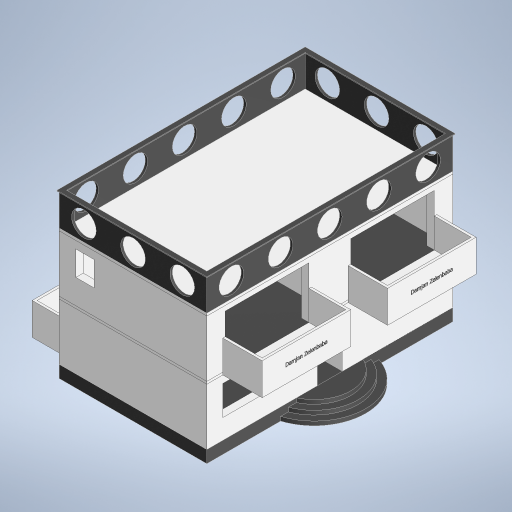
# Autodesk Inventor part: House
Saved by Autodesk Inventor 2024 (Build 280153000, 153)
## iProperties
Created: 2023-06-27
Part Number: House
Material: Generic
Document SubType Name: Modeling
Designer: 69
Density: 1 g/cm^3
Appearance: White
Author: 69
Autodesk Inventor part; units mm, degrees
(part 1 of 3)
ref_plane "YZ Plane" through (0, 0, 0) normal (1, 0, 0) x (0, 1, 0)
ref_plane "XZ Plane" through (0, 0, 0) normal (0, 1, 0) x (-1, 0, 0)
ref_plane "XY Plane" through (0, 0, 0) normal (0, 0, 1) x (1, 0, 0)
sketch "Sketch1" plane through (0, 0, 0) normal (0, 1, 0) x (-1, 0, 0)
  line L0 (3000, 5000) -> (-3000, 5000)
  line L1 (-3000, 5000) -> (-3000, -5000)
  line L2 (-3000, -5000) -> (3000, -5000)
  line L3 (3000, -5000) -> (3000, 5000)
  line L4 (3000, 5000) -> (-3000, -5000) construction
  line L5 (-3000, 5000) -> (3000, -5000) construction
  point P0 (0, 0)
  dimension "d0" = 6000
  dimension "d1" = 10000
  constraints: 12 end point, 2 midpoint, 2 parallel, 1 horizontal, 1 perpendicular
  measures "d0" distance of L2.end L1.end
  measures "d1" distance of L1.end L0.end
extrude "Extrusion1" add sketch "Sketch1" along normal blind 500
sketch "Sketch2" plane through (0, 500, 0) normal (0, 1, 0) x (1, 0, 0)
  line L0 (3000, -5000) -> (3000, 5000) projected
  line L1 (3000, 5000) -> (-3000, 5000) projected
  line L2 (-3000, 5000) -> (-3000, -5000) projected
  line L3 (-3000, -5000) -> (3000, -5000) projected
  line L4 (-2700, -4700) -> (-2700, 4700)
  line L5 (-2700, 4700) -> (2700, 4700)
  line L6 (2700, 4700) -> (2700, -4700)
  line L7 (2700, -4700) -> (-2700, -4700)
  line L8 (2700, 4700) -> (700, 4700)
  line L9 (700, 4700) -> (700, 600)
  line L10 (700, 500) -> (2700, 500)
  line L11 (2700, 500) -> (2700, 4700)
  line L12 (-2700, 4700) -> (600, 4700)
  line L13 (600, 4700) -> (600, 1000)
  line L14 (600, 1000) -> (-2700, 1000)
  line L15 (-2700, 1000) -> (-2700, 4700)
  line L16 (-2700, -4700) -> (-50, -4700)
  line L17 (-50, -4700) -> (-50, -1000)
  line L18 (-50, -1000) -> (-2700, -1000)
  line L19 (-2700, -1000) -> (-2700, -4700)
  line L20 (2700, -4700) -> (50, -4700)
  line L21 (50, -4700) -> (50, -600)
  line L22 (50, -500) -> (2700, -500)
  line L23 (2700, -500) -> (2700, -4700)
  line L24 (-1200, -1000) -> (-1200, 1000)
  line L25 (-2700, -900) -> (-50, -900)
  line L26 (-50, -900) -> (-50, -500)
  line L27 (-50, -500) -> (50, -500)
  line L28 (50, -600) -> (2700, -600)
  line L29 (-2700, 900) -> (600, 900)
  line L30 (600, 900) -> (600, 500)
  line L31 (600, 500) -> (700, 500)
  line L32 (700, 600) -> (2700, 600)
  line L33 (-1200, -50) -> (-1950, -50)
  line L34 (-1950, -50) -> (-1950, 50)
  line L35 (-1950, 50) -> (-1200, 50)
  line L36 (-1200, 50) -> (-1200, -50)
  point P0 (0, 0)
  point P1 (2700, 0)
  point P2 (-2700, 0)
  point P3 (0, -4700)
  point P4 (-1950, 0)
  point P5 (-1200, 0)
  point P6 (-1200, 0)
  point P7 (2700, -600)
  point P8 (50, -4700)
  point P9 (700, 4700)
  point P10 (-2700, -1000)
  point P11 (-50, -4700)
  dimension "d4" = 300
  dimension "d5" = 500
  dimension "d6" = 2000
  dimension "d7" = 1000
  dimension "d8" = 100
  dimension "d9" = 1000
  dimension "d10" = 50
  dimension "d11" = 50
  dimension "d12" = 500
  dimension "d13" = 1500
  dimension "d14" = 100
  dimension "d15" = 100
  dimension "d16" = 100
  dimension "d17" = 100
  dimension "d18" = 100
  dimension "d19" = 100
  dimension "d20" = 2000
  dimension "d21" = 100
  dimension "d22" = 750
  constraints: 66 end point, 13 perpendicular, 10 parallel, 7 point on line, 6 horizontal, 6 midpoint, 2 horizontal alignment, 3 other
  measures "d4" distance between parallel lines of L2 L4
  measures "d5" distance of L10.end point (2700, 0)
  measures "d6" distance of L10.start L10.end
  measures "d7" distance of L14.end point (-2700, 0)
  measures "d8" distance between parallel lines of L9 L13
  measures "d9" distance of point (-2700, 0) L18.end
  measures "d10" distance of point (0, -4700) L16.end
  measures "d11" distance of point (0, -4700) L20.end
  measures "d12" distance of point (2700, 0) L22.end
  measures "d13" distance between parallel lines of L4 L24
  measures "d14" distance between parallel lines of L22 L28
  measures "d15" distance between parallel lines of L21 L26
  measures "d16" distance between parallel lines of L18 L25
  measures "d17" distance between parallel lines of L32 L10
  measures "d18" distance between parallel lines of L9 L30
  measures "d19" distance between parallel lines of L14 L29
  measures "d20" distance between parallel lines of L6 L9
  measures "d21" distance of L33.end L34.end
  measures "d22" distance of L34.end L35.end
extrude "Extrusion2" add sketch "Sketch2" along normal blind 2400 separate body contours L3 L2 L1 L0 | L4 L25 L24 L18 | L17 L18 L24 L25 L26 L27 L22 L6 L28 L21 L7 | L4 L14 L24 L29 | L24 L14 L13 L5 L9 L32 L6 L10 L31 L30 L29 | L33 L34 L35 L24
sketch "Sketch3" plane through (3000, 500, 5000) normal (1, 0, 0) x (0, 0, -1)
  line L0 (0, 0) -> (10000, 0) projected
  line L1 (10000, 0) -> (10000, 2400) projected
  line L2 (0, 2400) -> (10000, 2400) projected
  line L3 (0, 0) -> (0, 2400) projected
  line L4 (0, 0) -> (10000, 0) projected
  line L5 (4500, 0) -> (5500, 0)
  line L6 (5500, 0) -> (5500, 2100)
  line L7 (5500, 2100) -> (4500, 2100)
  line L8 (4500, 2100) -> (4500, 0)
  point P0 (5000, -500)
  point P1 (5000, 0)
  point P2 (4400, 0)
  point P3 (5000, 0)
  dimension "d25" = 2100
  dimension "d26" = 1000
  constraints: 8 end point, 2 midpoint, 2 parallel, 1 coincident, 1 horizontal, 1 horizontal alignment, 1 perpendicular, 1 point on line
  measures "d25" distance of L5.end L6.end
  measures "d26" distance of L6.end L7.end
extrude "Extrusion3" cut sketch "Sketch3" against normal blind 500 contours L8 L7 L6 L0 bodies 2
sketch "Sketch4" plane through (2700, 500, -600) normal (0, 0, -1) x (-1, 0, 0)
  line L0 (1100, 2100) -> (1900, 2100)
  line L1 (1900, 2100) -> (1900, 0)
  line L2 (1900, 0) -> (1100, 0)
  line L3 (1100, 0) -> (1100, 2100)
  line L4 (2000, 0) -> (2000, 2400) projected
  line L5 (0, 0) -> (2000, 0) projected
  point P0 (2700, -500)
  dimension "d29" = 100
  dimension "d30" = 800
  dimension "d31" = 2100
  constraints: 8 end point, 2 parallel, 1 collinear, 1 horizontal, 1 perpendicular
  measures "d29" distance between parallel lines of L4 L1
  measures "d30" distance of L0.start L0.end
  measures "d31" distance of L2.end L0.start
extrude "Extrusion4" cut sketch "Sketch4" against normal blind 200 bodies 2
sketch "Sketch5" plane through (600, 500, -1000) normal (0, 0, -1) x (-1, 0, 0)
  line L0 (100, 2100) -> (900, 2100)
  line L1 (900, 2100) -> (900, 0)
  line L2 (900, 0) -> (100, 0)
  line L3 (100, 0) -> (100, 2100)
  line L4 (0, 0) -> (3300, 0) projected
  line L5 (0, 0) -> (0, 2400) projected
  point P0 (600, -500)
  dimension "d34" = 100
  dimension "d36" = 2100
  dimension "d37" = 800
  constraints: 8 end point, 2 parallel, 1 collinear, 1 horizontal, 1 perpendicular
  measures "d34" distance between parallel lines of L5 L3
  measures "d36" distance of L0.end L1.end
  measures "d37" distance of L0.start L0.end
extrude "Extrusion5" cut sketch "Sketch5" against normal blind 200 bodies 2
sketch "Sketch6" plane through (3000, 500, 500) normal (0, 0, -1) x (-1, 0, 0)
  line L0 (2050, 2100) -> (2850, 2100)
  line L1 (2850, 2100) -> (2850, 0)
  line L2 (2850, 0) -> (2050, 0)
  line L3 (2050, 0) -> (2050, 2100)
  line L4 (0, 0) -> (3050, 0) projected
  line L5 (3050, 0) -> (3050, 2400) projected
  point P0 (3000, -500)
  dimension "d40" = 800
  dimension "d41" = 2100
  dimension "d42" = 200
  constraints: 8 end point, 2 parallel, 1 collinear, 1 horizontal, 1 perpendicular
  measures "d40" distance of L0.start L0.end
  measures "d41" distance of L2.end L0.start
  measures "d42" distance between parallel lines of L5 L1
extrude "Extrusion6" cut sketch "Sketch6" against normal blind 200 bodies 2
sketch "Sketch8" plane through (0, 0, 0) normal (0, 1, 0) x (-1, 0, 0)
  line L0 (-3000, 5000) -> (-3000, -5000) projected
  line L1 (-3000, 5000) -> (-3000, -5000) projected
  arc A0 (-3000, 2000) -> (-3000, -2000) centre (-2359.6876, 0) ccw
  point P0 (0, 0)
  point P1 (-4459.6876, 0)
  point P2 (-3000, 0)
  point P3 (-3000, -2000)
  point P4 (-3000, 2000)
  dimension "d50" = 4000
  dimension "d62" = 2100
  constraints: 3 point on circle, 2 point on line, 1 centre point, 1 horizontal alignment, 1 midpoint
  measures "d50" distance of A0.end A0.start
  measures "d62" radius of A0
extrude "Extrusion8" add sketch "Sketch8" along normal blind 166.66 separate body
sketch "Sketch9" plane through (0, 166.66, 0) normal (0, 1, 0) x (1, 0, 0)
  arc A0 (3000, -2000) -> (3000, 2000) centre (2359.6876, 0) ccw projected
  arc A1 (3000, -1682.2604) -> (3000, 1682.2604) centre (2359.6876, 0) ccw
  line L0 (3000, -5000) -> (3000, 5000) projected
  point P0 (0, 0)
  point P1 (3000, 1135.7817)
  point P2 (3000, -1135.7817)
  dimension "d55" = 300
  constraints: 2 point on circle, 2 point on line, 1 centre point
  measures "d55" radial gap between concentric circles of A0 A1
extrude "Extrusion9" add sketch "Sketch9" along normal blind 166.66 contours L0 A1 bodies 3
sketch "Sketch10" plane through (0, 333.32, 0) normal (0, 1, 0) x (1, 0, 0)
  arc A0 (3000, -1682.2604) -> (3000, 1682.2604) centre (2359.6876, 0) ccw projected
  line L0 (3000, -5000) -> (3000, 5000) projected
  arc A1 (3000, -1356.466) -> (3000, 1356.466) centre (2359.6876, 0) ccw
  point P0 (0, 0)
  point P1 (3000, -1135.7817)
  point P2 (3000, 1135.7817)
  point P3 (3000, 714.1428)
  point P4 (3000, -714.1428)
  dimension "d58" = 300
  constraints: 2 point on circle, 2 point on line, 1 centre point
  measures "d58" radial gap between concentric circles of A0 A1
extrude "Extrusion10" add sketch "Sketch10" along normal up to surface (166.68 mm away) contours L0 A1 bodies 3
sketch "Sketch15" plane through (-1200, 500, 50) normal (1, 0, 0) x (0, 0, -1)
  line L0 (100, 0) -> (0, 0) projected
  line L1 (0, 0) -> (0, 2400) projected
  line L2 (100, 2400) -> (0, 2400) projected
  line L3 (100, 0) -> (100, 2400) projected
  point P0 (50, -500)
extrude "Extrusion12" add sketch "Sketch15" along normal blind 500 bodies 2
sketch "Sketch16" plane through (-1950, 500, -50) normal (0, 0, -1) x (-1, 0, 0)
  line L0 (-1250, 0) -> (750, 0)
  line L1 (1050, 0) -> (-4950, 0) projected
  line L2 (0, 0) -> (0, 2400) projected
  line L3 (-1250, 200) -> (750, 200)
  line L4 (-1250, 400) -> (750, 400)
  line L5 (-1250, 600) -> (750, 600)
  line L6 (-1250, 800) -> (750, 800)
  line L7 (-1250, 1000) -> (750, 1000)
  line L8 (-1250, 1200) -> (750, 1200)
  line L9 (-1250, 1400) -> (750, 1400)
  line L10 (-1250, 1600) -> (750, 1600)
  line L11 (-1250, 1800) -> (750, 1800)
  line L12 (-1250, 2000) -> (750, 2000)
  line L13 (-1250, 2200) -> (750, 2200)
  line L14 (-1000, 200) -> (-1000, 400)
  line L15 (-750, 400) -> (-750, 600)
  line L16 (-500, 600) -> (-500, 800)
  line L17 (-250, 800) -> (-250, 1000)
  line L18 (250, 1000) -> (-1000, 0)
  line L19 (-1250, 200) -> (-1250, 0)
  line L20 (750, 0) -> (750, 2400) projected
  point P0 (-1950, -500)
  point P1 (0, 200)
  point P2 (0, 400)
  point P3 (0, 600)
  point P4 (0, 800)
  point P5 (0, 1000)
  point P6 (0, 1200)
  point P7 (0, 1400)
  point P8 (0, 1600)
  point P9 (0, 1800)
  point P10 (0, 2000)
  point P11 (0, 2200)
  point P12 (-1000, 0)
  point P13 (0, 1200)
  point P14 (0, 1000)
  dimension "d91" = 200
  dimension "d96" = 250
  dimension "d97" = 250
  dimension "d98" = 250
  dimension "d99" = 250
  dimension "d100" = 250
  dimension "d101" = 250
  constraints: 36 end point, 8 point on line, 4 perpendicular, 2 midpoint, 2 vertical, 1 collinear, 45 other
  measures "d91" distance of L0.start L3.start
  measures "d96" distance of L3.start L14.start
  measures "d97" distance of L14.end L15.start
  measures "d98" distance of L16.start L15.end
  measures "d99" distance of L17.start L16.end
  measures "d100" distance of point (0, 1000) L18.start
  measures "d101" distance of L0.start L18.end
extrude "Extrusion13" add sketch "Sketch16" along normal blind 850 contours L19 L3 L18 L0 | L3 L14 L4 L18 | L4 L15 L5 L18 | L5 L16 L6 L18 | L6 L17 L7 L2 | L2 L7 L18 | L2 L8 L20 L7 bodies 2
sketch "Sketch17" plane through (0, 2900, 0) normal (0, 1, 0) x (1, 0, 0)
  line L0 (-1950, -50) -> (-700, -50) projected
  line L1 (-700, 50) -> (-700, -50) projected
  line L2 (-1950, 50) -> (-700, 50) projected
  line L3 (-1950, 50) -> (-1950, -50) projected
  point P0 (0, 0)
extrude "Extrusion14" cut sketch "Sketch17" against normal up to surface (2400 mm away) bodies 2
sketch "Sketch18" plane through (-1950, 500, -50) normal (0, 0, 1) x (1, 0, 0)
  line L0 (0, 1000) -> (0, 1200) projected
  line L1 (-750, 1200) -> (0, 1200) projected
  line L2 (-750, 1000) -> (-750, 1200) projected
  line L3 (-250, 1000) -> (-750, 1000) projected
  line L4 (-250, 1000) -> (1000, 0) projected
  line L5 (1250, 0) -> (1000, 0) projected
  line L6 (1250, 200) -> (1250, 0) projected
  line L7 (1250, 200) -> (1000, 200) projected
  line L8 (1000, 200) -> (1000, 400) projected
  line L9 (1000, 400) -> (750, 400) projected
  line L10 (750, 400) -> (750, 600) projected
  line L11 (750, 600) -> (500, 600) projected
  line L12 (500, 600) -> (500, 800) projected
  line L13 (500, 800) -> (250, 800) projected
  line L14 (250, 800) -> (250, 1000) projected
  line L15 (250, 1000) -> (0, 1000) projected
  point P0 (1950, -500)
extrude "Extrusion15" add sketch "Sketch18" along normal blind 50 bodies 2
sketch "Sketch19" plane through (-1950, 500, 0) normal (0, 0, 1) x (1, 0, 0)
  line L0 (1000, 200) -> (1000, 400) projected
  line L1 (1000, 400) -> (750, 400) projected
  line L2 (750, 400) -> (750, 600) projected
  line L3 (750, 600) -> (500, 600) projected
  line L4 (500, 600) -> (500, 800) projected
  line L5 (500, 800) -> (250, 800) projected
  line L6 (250, 800) -> (250, 1000) projected
  line L7 (250, 1000) -> (0, 1000) projected
  line L8 (0, 1000) -> (0, 1200) projected
  line L9 (0, 1200) -> (-750, 1200) projected
  line L10 (-750, 1000) -> (-750, 1200) projected
  line L11 (-750, 1000) -> (-250, 1000) projected
  line L12 (-250, 1000) -> (1000, 0) projected
  line L13 (1000, 0) -> (1250, 0) projected
  line L14 (1250, 0) -> (1250, 200) projected
  line L15 (1250, 200) -> (1000, 200) projected
  line L16 (-750, 1200) -> (0, 1200)
  line L17 (0, 1200) -> (0, 1000)
  line L18 (0, 1000) -> (-750, 1000)
  line L19 (-750, 1000) -> (-750, 1200)
  point P0 (1950, -500)
  constraints: 8 end point, 2 parallel, 1 horizontal, 1 perpendicular
extrude "Extrusion16" add sketch "Sketch19" along normal blind 900 contours L11 L10 L9 L8 L18 bodies 2
sketch "Sketch20" plane through (-50, 500, 900) normal (0, 0, -1) x (-1, 0, 0)
  line L0 (1900, 1200) -> (2650, 1200) projected
  line L1 (2650, 1200) -> (2650, 2400) projected
  line L2 (0, 2400) -> (2650, 2400) projected
  line L3 (0, 0) -> (0, 2400) projected
  line L4 (0, 1200) -> (2650, 1200)
  line L5 (0, 1400) -> (2650, 1400)
  line L6 (0, 1600) -> (2650, 1600)
  line L7 (0, 1800) -> (2650, 1800)
  line L8 (0, 2000) -> (2650, 2000)
  line L9 (0, 2200) -> (2650, 2200)
  line L10 (1900, 1200) -> (1900, 1400)
  line L11 (1650, 1400) -> (1650, 1600)
  line L12 (1400, 1600) -> (1400, 1800)
  line L13 (1150, 1800) -> (1150, 2000)
  line L14 (900, 2000) -> (900, 2200)
  line L15 (650, 2200) -> (650, 2400)
  line L16 (1650, 800) -> (1650, 1000) projected
  line L17 (1900, 1000) -> (1900, 1200) projected
  line L18 (1650, 1000) -> (1900, 1000) projected
  line L19 (1900, 1000) -> (150, 2400)
  point P0 (-50, -500)
  dimension "d112" = 200
  dimension "d117" = 250
  dimension "d118" = 250
  dimension "d119" = 250
  dimension "d120" = 250
  dimension "d121" = 250
  dimension "d122" = 500
  constraints: 26 end point, 13 point on line, 6 perpendicular, 1 collinear, 1 midpoint, 1 parallel, 1 vertical, 15 other
  measures "d112" distance of L4.start L5.start
  measures "d117" distance of L11.start L10.end
  measures "d118" distance of L12.start L11.end
  measures "d119" distance of L13.start L12.end
  measures "d120" distance of L14.start L13.end
  measures "d121" distance of L15.start L14.end
  measures "d122" distance of L19.end L15.end
extrude "Extrusion17" add sketch "Sketch20" along normal blind 900 contours L17 L19 L4 | L4 L19 L5 L10 | L19 L6 L11 L5 | L19 L7 L12 L6 | L19 L8 L13 L7 | L19 L9 L14 L8 | L19 L2 L15 L9 bodies 2
sketch "Sketch23" plane through (0, 2900, 0) normal (0, 1, 0) x (1, 0, 0)
  line L0 (3000, 5000) -> (-3000, 5000) projected
  line L1 (-3000, 5000) -> (-3000, -5000) projected
  line L2 (-3000, -5000) -> (3000, -5000) projected
  line L3 (3000, -5000) -> (3000, 5000) projected
  line L4 (-2700, 1000) -> (-2700, 4700) projected
  line L5 (-2700, 4700) -> (600, 4700) projected
  line L6 (600, 4700) -> (600, 1000) projected
  line L7 (600, 1000) -> (-2700, 1000) projected
  line L8 (-2700, 900) -> (600, 900) projected
  line L9 (600, 900) -> (600, 500) projected
  line L10 (600, 500) -> (2700, 500) projected
  line L11 (2700, 500) -> (2700, -500) projected
  line L12 (2700, -500) -> (-50, -500) projected
  line L13 (-50, -500) -> (-50, -900) projected
  line L14 (-50, -900) -> (-200, -900) projected
  line L15 (-200, -900) -> (-200, 0) projected
  line L16 (-700, 0) -> (-200, 0) projected
  line L17 (-700, -900) -> (-700, 0) projected
  line L18 (-700, -900) -> (-2700, -900) projected
  line L19 (-2700, -900) -> (-2700, 900) projected
  line L20 (2700, -600) -> (2700, -4700) projected
  line L21 (2700, -4700) -> (50, -4700) projected
  line L22 (50, -4700) -> (50, -600) projected
  line L23 (50, -600) -> (2700, -600) projected
  line L24 (700, 4700) -> (2700, 4700) projected
  line L25 (2700, 4700) -> (2700, 600) projected
  line L26 (2700, 600) -> (700, 600) projected
  line L27 (700, 600) -> (700, 4700) projected
  line L28 (-2700, -1000) -> (-50, -1000) projected
  line L29 (-50, -1000) -> (-50, -4700) projected
  line L30 (-50, -4700) -> (-2700, -4700) projected
  line L31 (-2700, -4700) -> (-2700, -1000) projected
  line L32 (-700, -900) -> (-200, -900)
  point P0 (0, 0)
  constraints: 2 end point, 1 perpendicular
extrude "Extrusion19" cut sketch "Sketch23" against normal blind 100 bodies 2
sketch "Sketch29" plane through (0, 2800, 0) normal (0, 1, 0) x (1, 0, 0)
  line L0 (50, -600) -> (50, -4700) projected
  line L1 (-50, -4700) -> (-50, -1000) projected
  line L2 (50, -4700) -> (-50, -4700)
  line L3 (-50, -1000) -> (50, -1000)
  point P0 (0, 0)
  constraints: 4 end point, 1 horizontal, 1 perpendicular, 1 point on line
extrude "Extrusion25" cut sketch "Sketch29" against normal up to surface (2300 mm away) bodies 2
sketch "Sketch30" plane through (0, 2800, 0) normal (0, 1, 0) x (1, 0, 0)
  line L0 (-3000, 5000) -> (-3000, -5000) projected
  line L1 (3000, -5000) -> (3000, 5000) projected
  line L2 (-3000, -5000) -> (3000, -5000)
  line L3 (3000, -5000) -> (3000, 5000)
  line L4 (3000, 5000) -> (-3000, 5000)
  line L5 (-3000, 5000) -> (-3000, -5000)
  line L6 (-2700, 900) -> (-2700, -900) projected
  line L7 (600, 900) -> (-2700, 900) projected
  line L8 (-2700, -900) -> (-200, -900)
  line L9 (-200, -900) -> (-200, 900)
  line L10 (-200, 900) -> (-2700, 900)
  line L11 (-2700, 900) -> (-2700, -900)
  line L12 (-200, -900) -> (-200, 0) projected
  point P0 (0, 0)
  constraints: 16 end point, 4 parallel, 2 horizontal, 2 perpendicular, 1 collinear, 1 point on line
extrude "Extrusion26" add sketch "Sketch30" along normal blind 100 separate body
sketch "Sketch31" plane through (0, 2900, 0) normal (0, 1, 0) x (1, 0, 0)
  line L0 (-3000, 5000) -> (-3000, -5000) projected
  line L1 (3000, -5000) -> (3000, 5000) projected
  line L2 (-3000, -5000) -> (3000, -5000)
  line L3 (3000, -5000) -> (3000, 5000)
  line L4 (3000, 5000) -> (-3000, 5000)
  line L5 (-3000, 5000) -> (-3000, -5000)
  line L6 (-2700, -4700) -> (-2700, -1000) projected
  line L7 (2700, 600) -> (2700, 4700) projected
  line L8 (-2700, -4700) -> (2700, -4700)
  line L9 (2700, -4700) -> (2700, 4700)
  line L10 (2700, 4700) -> (-2700, 4700)
  line L11 (-2700, 4700) -> (-2700, -4700)
  point P0 (0, 0)
  constraints: 16 end point, 4 parallel, 2 horizontal, 2 perpendicular
extrude "Extrusion27" add sketch "Sketch31" along normal blind 2300 separate body
sketch "Sketch32" plane through (0, 2900, 0) normal (0, 1, 0) x (1, 0, 0)
  line L0 (-2700, -4700) -> (-2700, 4700) projected
  line L1 (2700, -4700) -> (-2700, -4700) projected
  line L2 (2700, 4700) -> (2700, -4700) projected
  line L3 (-2700, 4700) -> (2700, 4700) projected
  line L4 (-2700, 900) -> (-200, 900) projected
  line L5 (-200, -900) -> (-2700, -900) projected
  line L6 (550, -900) -> (550, 900)
  line L7 (-200, -900) -> (-200, 0) projected
  line L8 (-200, 900) -> (-200, -900) projected
  line L9 (550, -900) -> (-200, -900)
  line L10 (550, 900) -> (-200, 900)
  line L11 (600, 900) -> (-2700, 900) projected
  line L12 (-2700, -1000) -> (650, -1000)
  line L13 (650, -1000) -> (650, 1000)
  line L14 (650, 1000) -> (-2700, 1000)
  line L15 (650, -50) -> (2700, -50)
  line L16 (650, 50) -> (2700, 50)
  line L17 (-1200, 1000) -> (-1200, 4700)
  line L18 (-1200, -1000) -> (-1200, -4700)
  line L19 (-1100, 1000) -> (-1100, 4700)
  line L20 (-1100, -1000) -> (-1100, -4700)
  point P0 (0, 0)
  dimension "d146" = 750
  dimension "d147" = 100
  dimension "d148" = 100
  dimension "d149" = 100
  dimension "d150" = 50
  dimension "d151" = 50
  dimension "d159" = 100
  dimension "d160" = 1500
  constraints: 24 end point, 18 point on line, 7 perpendicular, 2 horizontal alignment, 1 collinear, 1 horizontal, 1 vertical
  measures "d146" distance between parallel lines of L7 L6
  measures "d147" distance between parallel lines of L5 L12
  measures "d148" distance between parallel lines of L14 L4
  measures "d149" distance between parallel lines of L13 L6
  measures "d150" vertical distance of point (0, 0) L16.start
  measures "d151" distance from line of point (0, 0) L15
  measures "d159" distance between parallel lines of L19 L17
  measures "d160" distance between parallel lines of L0 L17
extrude "Extrusion28" add sketch "Sketch32" along normal blind 2300 contours L0 L5 L9 L6 L10 L4 L14 L13 L12 | L18 L12 L20 L1 | L15 L13 L16 L2 | L17 L3 L19 L14 bodies 4
sketch "Sketch33" plane through (550, 2900, -900) normal (-1, 0, 0) x (0, 0, 1)
  line L0 (50, 2100) -> (850, 2100)
  line L1 (850, 2100) -> (850, 0)
  line L2 (850, 0) -> (50, 0)
  line L3 (50, 0) -> (50, 2100)
  line L4 (950, 2100) -> (1750, 2100)
  line L5 (1750, 2100) -> (1750, 0)
  line L6 (1750, 0) -> (950, 0)
  line L7 (950, 0) -> (950, 2100)
  line L8 (850, 0) -> (850, 2300) projected
  line L9 (950, 0) -> (950, 2300) projected
  line L10 (-100, 0) -> (850, 0) projected
  point P0 (900, -2900)
  dimension "d154" = 2100
  dimension "d155" = 800
  dimension "d156" = 800
  constraints: 16 end point, 4 parallel, 3 collinear, 2 horizontal, 2 perpendicular, 2 point on line
  measures "d154" distance of L2.end L0.start
  measures "d155" distance of L0.start L0.end
  measures "d156" distance of L4.start L4.end
extrude "Extrusion29" cut sketch "Sketch33" against normal blind 100 bodies 4
sketch "Sketch34" plane through (-1100, 2900, 4700) normal (1, 0, 0) x (0, 0, -1)
  line L0 (2700, 2100) -> (3500, 2100)
  line L1 (3500, 2100) -> (3500, 0)
  line L2 (3500, 0) -> (2700, 0)
  line L3 (2700, 0) -> (2700, 2100)
  line L4 (5900, 2100) -> (6700, 2100)
  line L5 (6700, 2100) -> (6700, 0)
  line L6 (6700, 0) -> (5900, 0)
  line L7 (5900, 0) -> (5900, 2100)
  line L8 (3800, 0) -> (3800, 2300) projected
  line L9 (5600, 0) -> (5600, 2300) projected
  line L10 (0, 0) -> (3700, 0) projected
  point P0 (4700, -2900)
  dimension "d161" = 2100
  dimension "d162" = 2100
  dimension "d163" = 800
  dimension "d164" = 800
  dimension "d165" = 300
  dimension "d166" = 300
  constraints: 16 end point, 4 parallel, 2 horizontal, 2 perpendicular, 1 collinear, 1 point on line
  measures "d161" distance of L2.end L0.start
  measures "d162" distance of L6.end L4.start
  measures "d163" distance of L0.start L0.end
  measures "d164" distance of L4.start L4.end
  measures "d165" distance between parallel lines of L8 L1
  measures "d166" distance between parallel lines of L9 L7
extrude "Extrusion30" cut sketch "Sketch34" against normal blind 100 bodies 4
sketch "Sketch35" plane through (3000, 2900, 5000) normal (1, 0, 0) x (0, 0, -1)
  line L0 (300, 0) -> (300, 2300) projected
  line L1 (4100, 0) -> (5000, 0) projected
  line L2 (300, 2300) -> (4950, 2300)
  line L3 (4950, 2300) -> (4950, 0)
  line L4 (4950, 0) -> (300, 0)
  line L5 (300, 0) -> (300, 2300)
  line L6 (9700, 0) -> (9700, 2300) projected
  line L7 (5050, 2300) -> (9700, 2300)
  line L8 (9700, 2300) -> (9700, 0)
  line L9 (9700, 0) -> (5050, 0)
  line L10 (5050, 0) -> (5050, 2300)
  line L11 (4150, 0) -> (4150, 2100) projected
  line L12 (5850, 2100) -> (5850, 0) projected
  line L13 (5850, 2100) -> (9700, 2100)
  line L14 (4150, 2100) -> (300, 2100)
  line L15 (750, 2100) -> (750, 0)
  line L16 (0, 0) -> (0, 2300) projected
  line L17 (9250, 2100) -> (9250, 0)
  line L18 (10000, 0) -> (10000, 2300) projected
  point P0 (5000, -2900)
  dimension "d169" = 750
  dimension "d170" = 750
  constraints: 24 end point, 8 point on line, 4 parallel, 3 perpendicular, 2 horizontal, 2 vertical, 1 coincident
  measures "d169" distance between parallel lines of L16 L15
  measures "d170" distance between parallel lines of L18 L17
extrude "Extrusion31" cut sketch "Sketch35" against normal blind 300 contours L15 L14 L11 L1 L4 | L9 L12 L13 L17 bodies 5
sketch "Sketch36" plane through (3000, 2900, -5000) normal (0, 0, -1) x (-1, 0, 0)
  line L0 (5700, 0) -> (4200, 0) projected
  line L1 (5700, 0) -> (5700, 2300) projected
  line L2 (4200, 2300) -> (5700, 2300) projected
  line L3 (4200, 0) -> (4200, 2300) projected
  line L4 (4575, 2000) -> (5325, 2000)
  line L5 (5325, 2000) -> (5325, 1000)
  line L6 (5325, 1000) -> (4575, 1000)
  line L7 (4575, 1000) -> (4575, 2000)
  point P0 (3000, -2900)
  point P1 (4950, 2000)
  point P2 (4950, 2300)
  dimension "d173" = 750
  dimension "d174" = 1000
  dimension "d175" = 300
  constraints: 8 end point, 2 midpoint, 2 parallel, 1 horizontal, 1 perpendicular, 1 vertical alignment
  measures "d173" distance of L5.end L6.end
  measures "d174" distance of L4.end L5.end
  measures "d175" distance between parallel lines of L2 L4
extrude "Extrusion32" cut sketch "Sketch36" against normal blind 300 contours L4 L5 L6 L7 bodies 5
mirror "Mirror1" about plane through (0, 0, 0) normal (0, 0, 1) of "Extrusion32" bodies 5
sketch "Sketch38" plane through (3000, 2900, -5000) normal (1, 0, 0) x (0, 0, -1)
  line L0 (0, -100) -> (-10000, -100) projected
  line L1 (-9350, 1200) -> (-5750, 1200)
  line L2 (-5750, 1200) -> (-5750, -100)
  line L3 (-5750, -100) -> (-9350, -100)
  line L4 (-9350, -100) -> (-9350, 1200)
  line L5 (-9250, 0) -> (-9250, 2100) projected
  line L6 (-5850, 2100) -> (-5850, 0) projected
  line L7 (-10000, 0) -> (0, 0) projected
  point P0 (-5000, -2900)
  point P1 (-9350, -100)
  dimension "d187" = 100
  dimension "d188" = 100
  dimension "d189" = 1200
  constraints: 8 end point, 2 parallel, 1 horizontal, 1 perpendicular, 1 point on line
  measures "d187" distance between parallel lines of L5 L4
  measures "d188" distance between parallel lines of L6 L2
  measures "d189" distance between parallel lines of L7 L1
extrude "Extrusion34" add sketch "Sketch38" along normal blind 1600 separate body
sketch "Sketch39" plane through (3000, 4100, 4350) normal (0, 1, 0) x (1, 0, 0)
  line L0 (0, 3600) -> (0, 0) projected
  line L1 (0, 0) -> (1600, 0) projected
  line L2 (1600, 3600) -> (1600, 0) projected
  line L3 (0, 3600) -> (1600, 3600) projected
  line L4 (0, 100) -> (1500, 100)
  line L5 (1500, 100) -> (1500, 3500)
  line L6 (1500, 3500) -> (0, 3500)
  point P0 (-3000, 4350)
  dimension "d192" = 100
  dimension "d193" = 100
  dimension "d194" = 100
  constraints: 6 end point, 2 perpendicular, 2 point on line, 1 parallel
  measures "d192" distance between parallel lines of L3 L6
  measures "d193" distance between parallel lines of L2 L5
  measures "d194" distance between parallel lines of L1 L4
extrude "Extrusion35" cut sketch "Sketch39" against normal blind 1200 contours L6 L5 L4 L0 bodies 6
mirror "Mirror2" about plane through (0, 0, 0) normal (0, 0, 1) of "Extrusion34", "Extrusion35" bodies 6
sketch "Sketch40" plane through (3000, 500, 5000) normal (1, 0, 0) x (0, 0, -1)
  line L0 (650, 2000) -> (3000, 2000)
  line L1 (3000, 2000) -> (3000, 800)
  line L2 (3000, 800) -> (650, 800)
  line L3 (650, 800) -> (650, 2000)
  line L4 (650, 2300) -> (4250, 2300) projected
  point P0 (5000, -500)
  point P1 (3000, -333.34)
  dimension "d197" = 1200
  dimension "d198" = 300
  constraints: 8 end point, 2 parallel, 2 vertical alignment, 1 horizontal, 1 perpendicular
  measures "d197" distance of L2.end L0.start
  measures "d198" distance between parallel lines of L4 L0
extrude "Extrusion36" cut sketch "Sketch40" against normal blind 300 bodies 2
sketch "Sketch41" plane through (3000, 500, -5000) normal (0, 0, -1) x (-1, 0, 0)
  line L0 (925, 2000) -> (1675, 2000)
  line L1 (1675, 2000) -> (1675, 1000)
  line L2 (1675, 1000) -> (925, 1000)
  line L3 (925, 1000) -> (925, 2000)
  line L4 (2300, 2300) -> (300, 2300) projected
  point P0 (3000, -500)
  point P1 (1300, 2000)
  point P2 (1300, 2300)
  dimension "d201" = 750
  dimension "d202" = 1000
  dimension "d203" = 300
  constraints: 8 end point, 2 midpoint, 2 parallel, 1 horizontal, 1 perpendicular, 1 vertical alignment
  measures "d201" distance of L1.end L2.end
  measures "d202" distance of L0.end L1.end
  measures "d203" distance between parallel lines of L4 L0
extrude "Extrusion37" cut sketch "Sketch41" against normal blind 300 bodies 2
sketch "Sketch42" plane through (3000, 500, -5000) normal (0, 0, -1) x (-1, 0, 0)
  line L0 (2400, 2300) -> (5700, 2300) projected
  line L1 (2550, 2000) -> (5550, 2000)
  line L2 (5550, 2000) -> (5550, 800)
  line L3 (5550, 800) -> (2550, 800)
  line L4 (2550, 800) -> (2550, 2000)
  point P0 (3000, -500)
  point P1 (4050, 2000)
  point P2 (4050, 2300)
  point P3 (1675, 2000)
  dimension "d206" = 3000
  dimension "d207" = 1200
  constraints: 8 end point, 2 midpoint, 2 parallel, 1 horizontal, 1 horizontal alignment, 1 perpendicular, 1 vertical alignment
  measures "d206" distance of L2.end L3.end
  measures "d207" distance of L1.end L2.end
extrude "Extrusion38" cut sketch "Sketch42" against normal blind 300 bodies 2
sketch "Sketch43" plane through (-3000, 500, -5000) normal (-1, 0, 0) x (0, 0, 1)
  line L0 (6000, 0) -> (6000, 2300) projected
  line L1 (9700, 0) -> (9700, 2300) projected
  line L2 (0, 0) -> (10000, 0) projected
  line L3 (6300, 2100) -> (9400, 2100)
  line L4 (9400, 2100) -> (9400, 0)
  line L5 (9400, 0) -> (6300, 0)
  line L6 (6300, 0) -> (6300, 2100)
  point P0 (5000, -500)
  point P1 (6300, 0)
  dimension "d210" = 300
  dimension "d211" = 300
  dimension "d212" = 2100
  constraints: 8 end point, 2 parallel, 1 horizontal, 1 perpendicular, 1 point on line
  measures "d210" distance between parallel lines of L0 L6
  measures "d211" distance between parallel lines of L1 L4
  measures "d212" distance of L3.end L4.end
extrude "Extrusion39" cut sketch "Sketch43" against normal blind 300 bodies 2
sketch "Sketch44" plane through (-3000, 0, -5000) normal (-1, 0, 0) x (0, 0, 1)
  line L0 (6200, 1700) -> (9500, 1700)
  line L1 (9500, 1700) -> (9500, 400)
  line L2 (9500, 400) -> (6200, 400)
  line L3 (6200, 400) -> (6200, 1700)
  line L4 (9400, 2600) -> (9400, 500) projected
  line L5 (0, 500) -> (10000, 500) projected
  line L6 (6300, 500) -> (6300, 2600) projected
  point P0 (5000, 0)
  dimension "d215" = 100
  dimension "d216" = 100
  dimension "d217" = 100
  dimension "d218" = 1300
  constraints: 8 end point, 2 parallel, 1 horizontal, 1 perpendicular
  measures "d215" distance between parallel lines of L4 L1
  measures "d216" distance between parallel lines of L2 L5
  measures "d217" distance between parallel lines of L6 L3
  measures "d218" distance between parallel lines of L2 L0
extrude "Extrusion40" add sketch "Sketch44" along normal blind 1600 separate body
sketch "Sketch46" plane through (-3000, 1700, 4500) normal (0, 1, 0) x (1, 0, 0)
  line L0 (0, 0) -> (0, 3300) projected
  line L1 (0, 3300) -> (-1600, 3300) projected
  line L2 (-1600, 0) -> (-1600, 3300) projected
  line L3 (0, 0) -> (-1600, 0) projected
  line L4 (0, 3200) -> (-1500, 3200)
  line L5 (-1500, 3200) -> (-1500, 100)
  line L6 (-1500, 100) -> (0, 100)
  line L7 (0, 100) -> (0, 3200)
  line L8 (0, 9500) -> (0, -500) projected
  point P0 (3000, 4500)
  point P1 (0, 100)
  point P2 (0, 3200)
  dimension "d226" = 100
  dimension "d227" = 100
  dimension "d228" = 100
  constraints: 8 end point, 2 parallel, 1 collinear, 1 horizontal, 1 perpendicular
  measures "d226" distance between parallel lines of L2 L5
  measures "d227" distance between parallel lines of L3 L6
  measures "d228" distance between parallel lines of L1 L4
extrude "Extrusion42" cut sketch "Sketch46" against normal blind 1200 contours L6 L5 L4 L0 bodies 7
sketch "Sketch47" plane through (-3000, 500, 5000) normal (-1, 0, 0) x (0, 0, 1)
  line L0 (-9350, 2000) -> (-6350, 2000)
  line L1 (-6350, 2000) -> (-6350, 800)
  line L2 (-6350, 800) -> (-9350, 800)
  line L3 (-9350, 800) -> (-9350, 2000)
  line L4 (-9700, 2300) -> (-6000, 2300) projected
  point P0 (-5000, -500)
  point P1 (-7850, 2000)
  point P2 (-7850, 2300)
  dimension "d231" = 300
  dimension "d232" = 3000
  dimension "d233" = 1200
  constraints: 8 end point, 2 midpoint, 2 parallel, 1 horizontal, 1 perpendicular, 1 vertical alignment
  measures "d231" distance between parallel lines of L4 L0
  measures "d232" distance of L0.start L0.end
  measures "d233" distance of L2.end L0.start
extrude "Extrusion43" cut sketch "Sketch47" against normal blind 300 bodies 2
sketch "Sketch51" plane through (0, 5200, 0) normal (0, 1, 0) x (1, 0, 0)
  line L0 (-3000, 5000) -> (-3000, -5000) projected
  line L1 (3000, -5000) -> (3000, 5000) projected
  line L2 (-3000, -5000) -> (3000, -5000)
  line L3 (3000, -5000) -> (3000, 5000)
  line L4 (3000, 5000) -> (-3000, 5000)
  line L5 (-3000, 5000) -> (-3000, -5000)
  point P0 (0, 0)
  constraints: 8 end point, 2 parallel, 1 horizontal, 1 perpendicular
extrude "Extrusion46" add sketch "Sketch51" along normal blind 100 separate body
sketch "Sketch52" plane through (0, 5300, 0) normal (0, 1, 0) x (1, 0, 0)
  line L0 (3000, -5000) -> (3000, 5000) projected
  line L1 (3000, 5000) -> (-3000, 5000) projected
  line L2 (-3000, 5000) -> (-3000, -5000) projected
  line L3 (-3000, -5000) -> (3000, -5000) projected
  line L4 (-2900, -4900) -> (-2900, 4900)
  line L5 (-2900, 4900) -> (2900, 4900)
  line L6 (2900, 4900) -> (2900, -4900)
  line L7 (2900, -4900) -> (-2900, -4900)
  point P0 (0, 0)
  dimension "d248" = 100
  constraints: 8 end point, 3 other
  measures "d248" distance between parallel lines of L2 L4
extrude "Extrusion47" add sketch "Sketch52" along normal blind 1300 separate body
sketch "Sketch53" plane through (3000, 5300, 5000) normal (1, 0, 0) x (0, 0, -1)
  circle A0 centre (1000, 650) radius 500
  line L0 (0, 0) -> (0, 1300) projected
  line L1 (0, 1300) -> (10000, 1300) projected
  line L2 (0, 0) -> (10000, 0) projected
  line L3 (10000, 0) -> (10000, 1300) projected
  circle A1 centre (3000, 650) radius 500
  circle A2 centre (5000, 650) radius 500
  circle A3 centre (7000, 650) radius 500
  circle A4 centre (9000, 650) radius 500
  point P0 (5000, -5300)
  point P1 (0, 650)
  point P2 (0, 650)
  dimension "d251" = 1000
  dimension "d252" = 1000
  dimension "d264" = 2000
  constraints: 5 centre point, 2 midpoint, 1 horizontal, 1 horizontal alignment, 8 other
  measures "d251" diameter of A0
  measures "d252" distance of A0.centre point (0, 650)
  measures "d264" distance of A0.centre A1.centre
extrude "Extrusion48" cut sketch "Sketch53" against normal blind 6000 contours A0 | A1 | A2 | A3 | A4 bodies 9
sketch "Sketch54" plane through (3000, 5300, -5000) normal (0, 0, -1) x (-1, 0, 0)
  circle A0 centre (1000, 650) radius 500
  line L0 (0, 0) -> (0, 1300) projected
  line L1 (0, 0) -> (6000, 0) projected
  line L2 (6000, 0) -> (6000, 1300) projected
  circle A1 centre (3000, 650) radius 500
  circle A2 centre (5000, 650) radius 500
  point P0 (3000, -5300)
  point P1 (0, 650)
  point P2 (0, 650)
  dimension "d269" = 1000
  dimension "d270" = 1000
  dimension "d273" = 2000
  constraints: 3 centre point, 2 midpoint, 1 horizontal, 1 horizontal alignment, 4 other
  measures "d269" diameter of A0
  measures "d270" distance of point (0, 650) A0.centre
  measures "d273" distance of A0.centre A1.centre
extrude "Extrusion49" cut sketch "Sketch54" against normal up to surface (10000 mm away) bodies 9
sketch "Sketch55" plane through (3000, 5300, -5000) normal (0, 0, -1) x (-1, 0, 0)
  line L0 (5900, 1300) -> (100, 1300) projected
  line L1 (-50, 1330) -> (150, 1330)
  line L2 (150, 1330) -> (150, 1300)
  line L3 (150, 1300) -> (-50, 1300)
  line L4 (-50, 1300) -> (-50, 1330)
  point P0 (3000, -5300)
  point P1 (0, 1300)
  dimension "d280" = 30
  dimension "d281" = 200
  dimension "d282" = 50
  constraints: 8 end point, 2 parallel, 1 horizontal, 1 perpendicular, 1 point on line
  measures "d280" distance of L3.end L1.start
  measures "d281" distance of L1.start L1.end
  measures "d282" distance of L3.end point (0, 1300)
sketch "Sketch56" plane through (0, 6600, 0) normal (0, 1, 0) x (1, 0, 0)
  line L0 (3000, 5000) -> (-3000, 5000) projected
  line L1 (-3000, 5000) -> (-3000, -5000) projected
  line L2 (-3000, -5000) -> (3000, -5000) projected
  line L3 (3000, -5000) -> (3000, 5000) projected
  line L4 (-2900, -4900) -> (-2900, 4900) projected
  line L5 (-2900, 4900) -> (2900, 4900) projected
  line L6 (2900, 4900) -> (2900, -4900) projected
  line L7 (2900, -4900) -> (-2900, -4900) projected
  point P0 (0, 0)
sweep "Sweep1" add profiles "Sketch55" path "Sketch56" bodies 9 path curves L3 L2 L1 L0